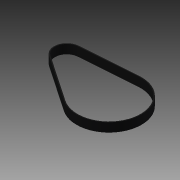
# Autodesk Inventor part: belt
Saved by Autodesk Inventor 2014 (Build 180170000, 170)
## iProperties
Created: 2014-05-23
Part Number: belt
Material: Generic
Document SubType Name: Modeling
Designer: brent
Density: 1 g/cm^3
Appearance: Default
Author: brent
Autodesk Inventor part; units mm, degrees
ref_plane "YZ Plane" through (0, 0, 0) normal (1, 0, 0) x (0, 1, 0)
ref_plane "XZ Plane" through (0, 0, 0) normal (0, 1, 0) x (-1, 0, 0)
ref_plane "XY Plane" through (0, 0, 0) normal (0, 0, 1) x (1, 0, 0)
derived "mountsketch_alt.ipt"
sketch "Sketch1" plane through (0, 0, 0) normal (0, 1, 0) x (-1, 0, 0)
  arc A0 (-19.7287, 38.1521) -> (-35.2875, -19.9218) centre (-37.6152, 11.823) ccw
  arc A1 (21.7165, -15.742) -> (27.5504, 6.0334) centre (20.8437, -3.839) ccw
  line L0 (-19.1548, 38.9712) -> (28.103, 6.8366)
  line L1 (27.5504, 6.0334) -> (-19.7287, 38.1521)
  line L2 (21.7165, -15.742) -> (-35.2875, -19.9218)
  arc A2 (21.7934, -16.7139) -> (28.103, 6.8366) centre (20.8437, -3.839) ccw
  line L3 (-35.2, -20.9181) -> (21.7934, -16.7139)
  arc A3 (-19.1548, 38.9712) -> (-35.2, -20.9181) centre (-37.6152, 11.823) ccw
  point P0 (0, 0)
  dimension "d1" = 63.66
  dimension "d4" = 23.87
  dimension "d8" = 60.5206
  constraints: 8 end point, 8 point on circle, 8 tangent, 4 centre point, 2 coincident
  measures "d1" diameter of A0
  measures "d4" diameter of A1
  measures "d8" distance of A1.centre A0.centre
extrude "Extrusion1" add sketch "Sketch1" along normal blind 9
equation "\"d1\" = largepulley_diameter"
equation "\"d4\" = smallpulley_diameter"
equation "\"d8\" = center_to_center_distance"
equation "\"largepulley_diameter\" = 63.66"
equation "\"smallpulley_diameter\" = 23.87"
equation "\"center_to_center_distance\" = 60.52058"
body "Solid1"
